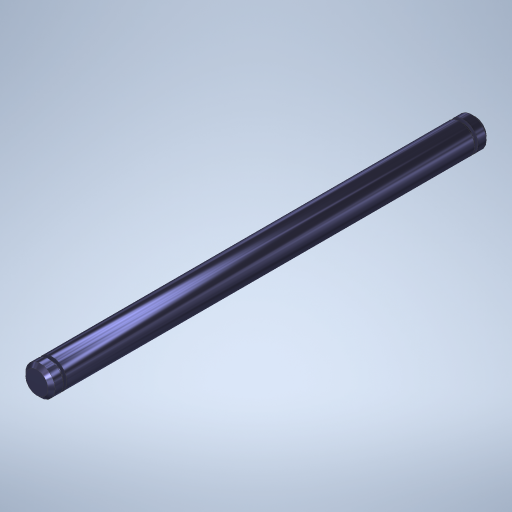
# Autodesk Inventor part: Front Lower Hinge Pin
Saved by Autodesk Inventor 2023.1 (Build 271208000, 208)
## iProperties
Created: 2019-11-29
Part Number: Front Lower Hinge Pin
Material: Generic
Document SubType Name: Modeling
Designer: Jopa
Density: 1 g/cm^3
Appearance: Default
Author: Jopa
Autodesk Inventor part; units mm, degrees
ref_plane "YZ Plane" through (0, 0, 0) normal (1, 0, 0) x (0, 1, 0)
ref_plane "XZ Plane" through (0, 0, 0) normal (0, 1, 0) x (-1, 0, 0)
ref_plane "XY Plane" through (0, 0, 0) normal (0, 0, 1) x (1, 0, 0)
sketch "Sketch1" plane through (0, 0, 0) normal (0, 0, 1) x (1, 0, 0)
  circle A0 centre (0, 0) radius 1.5875
  dimension "d0" = 3.175
  constraints: 1 centre point, 1 coincident
  measures "d0" diameter of A0
extrude "Extrusion1" add sketch "Sketch1" along normal mid plane 43.7845
sketch "Sketch2" plane through (0, 0, 21.8923) normal (0, 0, 1) x (1, 0, 0)
  circle A0 centre (0, 0) radius 1.1913
  dimension "d3" = 2.3825
  constraints: 1 centre point, 1 coincident
  measures "d3" diameter of A0
extrude "Extrusion2" add sketch "Sketch2" along normal blind 0.381
sketch "Sketch3" plane through (0, 0, 22.2733) normal (0, 0, 1) x (1, 0, 0)
  circle A0 centre (0, 0) radius 1.5875 projected
extrude "Extrusion3" add sketch "Sketch3" along normal blind 1.27
chamfer "Chamfer1" distance 0.381 angle 45 1 edges at (-1.5875, 0, 23.5433)
mirror "Mirror1" about plane through (0, 0, 0) normal (0, 0, 1) of "Extrusion2", "Extrusion3", "Chamfer1"
body "Solid1"
